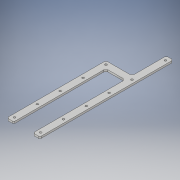
# Autodesk Inventor part: bar_-BattPow
Saved by Autodesk Inventor 2019 (Build 230136000, 136)
## iProperties
Created: 2019-05-08
Part Number: bar_-BattPow
Material: Ogólny
Document SubType Name: Modeling
Designer: Kurat
Density: 1 g/cm^3
Appearance: Domyślna
Author: Kurat
Autodesk Inventor part; units mm, degrees
ref_plane "YZ Plane" through (0, 0, 0) normal (1, 0, 0) x (0, 1, 0)
ref_plane "XZ Plane" through (0, 0, 0) normal (0, 1, 0) x (-1, 0, 0)
ref_plane "XY Plane" through (0, 0, 0) normal (0, 0, 1) x (1, 0, 0)
sketch "Szkic1" plane through (0, 0, 0) normal (0, 1, 0) x (-1, 0, 0)
  line L0 (38.1, 143.51) -> (30.48, 143.51)
  line L1 (27.94, 140.97) -> (27.94, 2.54)
  line L2 (25.4, 0) -> (2.54, 0)
  line L3 (0, 2.54) -> (0, 140.97)
  line L4 (-2.54, 143.51) -> (-10.16, 143.51)
  line L5 (-12.7, 140.97) -> (-12.7, -63.5)
  line L6 (-10.16, -66.04) -> (-2.54, -66.04)
  line L7 (0, -63.5) -> (0, -15.24)
  line L8 (2.54, -12.7) -> (38.1, -12.7)
  line L9 (40.64, -10.16) -> (40.64, 140.97)
  line L10 (34.29, 143.51) -> (34.29, -12.7) construction
  line L11 (-6.35, -66.04) -> (-6.35, 143.51) construction
  circle A0 centre (34.29, -6.35) radius 1.6
  circle A1 centre (-6.35, -6.35) radius 1.6
  circle A2 centre (34.29, 29.21) radius 1.6
  circle A3 centre (-6.35, 29.21) radius 1.6
  circle A4 centre (34.29, 64.77) radius 1.6
  circle A5 centre (-6.35, 64.77) radius 1.6
  circle A6 centre (34.29, 100.33) radius 1.6
  circle A7 centre (-6.35, 100.33) radius 1.6
  circle A8 centre (34.29, 135.89) radius 1.6
  circle A9 centre (-6.35, 135.89) radius 1.6
  circle A10 centre (-6.35, -58.42) radius 1.6
  line L12 (40.64, -10.16) -> (38.1, -12.7)
  line L13 (25.4, 0) -> (27.94, 2.54)
  line L14 (2.54, -12.7) -> (0, -15.24)
  line L15 (0, 2.54) -> (2.54, 0)
  line L16 (-2.54, -66.04) -> (0, -63.5)
  line L17 (-10.16, -66.04) -> (-12.7, -63.5)
  line L18 (-2.54, 143.51) -> (0, 140.97)
  line L19 (-10.16, 143.51) -> (-12.7, 140.97)
  line L20 (27.94, 140.97) -> (30.48, 143.51)
  line L21 (38.1, 143.51) -> (40.64, 140.97)
  line L22 (19.05, 0) -> (19.05, -6.35) construction
  line L23 (19.05, -6.35) -> (19.05, -12.7) construction
  line L24 (19.05, -6.35) -> (34.29, -6.35) construction
  line L25 (19.05, -6.35) -> (-6.35, -6.35) construction
  line L26 (39.64, 140.5558) -> (37.6858, 142.51)
  line L27 (37.6858, 142.51) -> (30.8942, 142.51)
  line L28 (30.8942, 142.51) -> (28.94, 140.5558)
  line L29 (28.94, 140.5558) -> (28.94, 2.1258)
  line L30 (28.94, 2.1258) -> (25.8142, -1)
  line L31 (25.8142, -1) -> (2.1258, -1)
  line L32 (2.1258, -1) -> (-1, 2.1258)
  line L33 (-1, 2.1258) -> (-1, 140.5558)
  line L34 (-1, 140.5558) -> (-2.9542, 142.51)
  line L35 (-2.9542, 142.51) -> (-9.7458, 142.51)
  line L36 (-9.7458, 142.51) -> (-11.7, 140.5558)
  line L37 (-11.7, 140.5558) -> (-11.7, -63.0858)
  line L38 (-11.7, -63.0858) -> (-9.7458, -65.04)
  line L39 (-9.7458, -65.04) -> (-2.9542, -65.04)
  line L40 (-2.9542, -65.04) -> (-1, -63.0858)
  line L41 (-1, -63.0858) -> (-1, -14.8258)
  line L42 (-1, -14.8258) -> (2.1258, -11.7)
  line L43 (2.1258, -11.7) -> (37.6858, -11.7)
  line L44 (37.6858, -11.7) -> (39.64, -9.7458)
  line L45 (39.64, -9.7458) -> (39.64, 140.5558)
  point P0 (0, 0)
  point P1 (40.64, 143.51)
  point P2 (27.94, 143.51)
  point P3 (27.94, 0)
  point P4 (0, 0)
  point P5 (0, 143.51)
  point P6 (-12.7, 143.51)
  point P7 (-12.7, -66.04)
  point P8 (0, -66.04)
  point P9 (0, -12.7)
  point P10 (40.64, -12.7)
  dimension "d0" = 12.7
  dimension "d1" = 209.55
  dimension "d2" = 156.21
  dimension "d3" = 27.94
  dimension "d4" = 3.2
  dimension "d5" = 3.2
  dimension "d8" = 35.56
  dimension "d13" = 3.2
  dimension "d14" = 7.62
  dimension "d16" = 2.54
  dimension "d17" = 2.54
  dimension "d18" = 2.54
  dimension "d19" = 2.54
  dimension "d20" = 2.54
  dimension "d21" = 2.54
  dimension "d22" = 2.54
  dimension "d23" = 2.54
  dimension "d24" = 2.54
  dimension "d25" = 2.54
  dimension "d26" = 2.54
  dimension "d27" = 2.54
  dimension "d28" = 2.54
  dimension "d29" = 2.54
  dimension "d30" = 2.54
  dimension "d31" = 2.54
  dimension "d32" = 2.54
  dimension "d33" = 2.54
  dimension "d34" = 2.54
  dimension "d35" = 2.54
  dimension "d36" = 12.7
  dimension "d37" = 1
  constraints: 92 end point, 33 point on line, 19 perpendicular, 11 centre point, 3 coincident, 3 midpoint, 2 equal length, 1 horizontal, 1 vertical, 35 other
  measures "d0" distance between parallel lines of L5 L7
  measures "d1" distance between parallel lines of L6 L4
  measures "d2" distance between parallel lines of L8 L0
  measures "d3" distance between parallel lines of L1 L3
  measures "d4" diameter of A0
  measures "d5" diameter of A1
  measures "d8" distance of A0.centre A2.centre
  measures "d13" diameter of A10
  measures "d14" distance from line of A10.centre L6
  measures "d16" distance of L9.start point (40.64, -12.7)
  measures "d17" distance of L8.end point (40.64, -12.7)
  measures "d18" distance of L2.start point (27.94, 0)
  measures "d19" distance of L1.end point (27.94, 0)
  measures "d20" distance of L8.start point (0, -12.7)
  measures "d21" distance of L7.end point (0, -12.7)
  measures "d22" distance of L3.start point (0, 0)
  measures "d23" distance of L2.end point (0, 0)
  measures "d24" distance of L6.end point (0, -66.04)
  measures "d25" distance of L7.start point (0, -66.04)
  measures "d26" distance of L6.start point (-12.7, -66.04)
  measures "d27" distance of L5.end point (-12.7, -66.04)
  measures "d28" distance of L4.start point (0, 143.51)
  measures "d29" distance of L3.end point (0, 143.51)
  measures "d30" distance of L4.end point (-12.7, 143.51)
  measures "d31" distance of L5.start point (-12.7, 143.51)
  measures "d32" distance of L1.start point (27.94, 143.51)
  measures "d33" distance of L0.end point (27.94, 143.51)
  measures "d34" distance of L0.start point (40.64, 143.51)
  measures "d35" distance of L9.end point (40.64, 143.51)
  measures "d36" distance between parallel lines of L8 L2
  measures "d37" distance between parallel lines of L9 L45
sketch "Szkic2" plane through (0, 0, 0) normal (0, 1, 0) x (-1, 0, 0)
  point P0 (0, 0)
extrude "Wyciągnięcie proste1" add sketch "Szkic1" along normal blind 3 contours L45 L44 L43 L42 L41 L40 L39 L38 L37 L36 L35 L34 L33 L32 L31 L30 L29 L28 L27 L26
equation "\"d17\" = d16"
equation "\"d18\" = d16"
equation "\"d19\" = d18"
equation "\"d20\" = d16"
equation "\"d21\" = d20"
equation "\"d22\" = d16"
equation "\"d23\" = d22"
equation "\"d24\" = d16"
equation "\"d25\" = d24"
equation "\"d26\" = d16"
equation "\"d27\" = d26"
equation "\"d28\" = d16"
equation "\"d29\" = d28"
equation "\"d30\" = d16"
equation "\"d31\" = d30"
equation "\"d32\" = d16"
equation "\"d33\" = d32"
equation "\"d34\" = d16"
equation "\"d35\" = d34"
